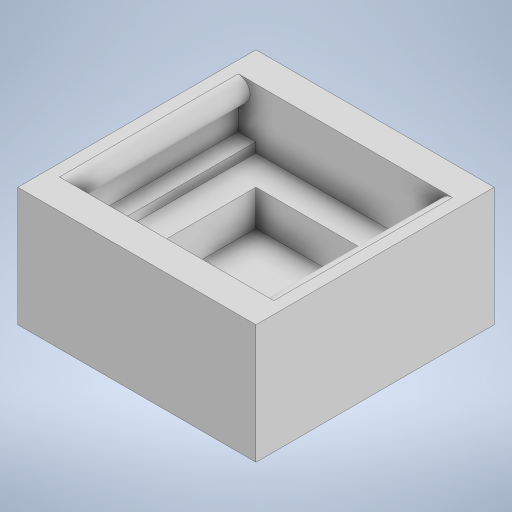
# Autodesk Inventor part: boxtest
Saved by Autodesk Inventor 2023 (Build 270158000, 158)
## iProperties
Created: 2022-12-05
Part Number: boxtest
Material: Generic
Document SubType Name: Modeling
Designer: spfow
Density: 1 g/cm^3
Appearance: Default
Author: spfow
Autodesk Inventor part; units mm, degrees
ref_plane "YZ Plane" through (0, 0, 0) normal (1, 0, 0) x (0, 1, 0)
sketch "Sketch1" plane through (0, 0, 0) normal (0, 1, 0) x (-1, 0, 0)
  line L0 (0, 0) -> (25.4, 0)
  line L1 (25.4, 0) -> (25.4, -25.4)
  line L2 (25.4, -25.4) -> (0, -25.4)
  line L3 (0, -25.4) -> (0, 0)
  dimension "d0" = 25.4
  dimension "d1" = 25.4
  constraints: 8 end point, 2 parallel, 1 horizontal, 1 perpendicular
  measures "d0" distance of L1.end L2.end
  measures "d1" distance of L0.end L1.end
extrude "Extrusion1" add sketch "Sketch1" along normal blind 12.7
shell "Shell1" thickness 6.35 removed faces 1 at (-8.4667, 12.7, -8.4667)
sketch "Sketch2" plane through (0, 12.7, 0) normal (0, 1, 0) x (1, 0, 0)
  line L0 (-22.225, 22.225) -> (-3.175, 22.225)
  line L1 (-3.175, 22.225) -> (-3.175, 3.175)
  line L2 (-3.175, 3.175) -> (-22.225, 3.175)
  line L3 (-22.225, 3.175) -> (-22.225, 22.225)
  line L4 (0, 0) -> (0, 25.4) projected
  line L5 (0, 25.4) -> (-25.4, 25.4) projected
  line L6 (-19.05, 19.05) -> (-6.35, 19.05) projected
  line L7 (-6.35, 19.05) -> (-6.35, 6.35) projected
  line L8 (-19.05, 19.05) -> (-6.35, 19.05)
  line L9 (-6.35, 19.05) -> (-6.35, 6.35)
  line L10 (-6.35, 6.35) -> (-19.05, 6.35)
  line L11 (-19.05, 6.35) -> (-19.05, 19.05)
  dimension "d5" = 19.05
  dimension "d6" = 19.05
  dimension "d7" = 3.175
  dimension "d8" = 3.175
  constraints: 16 end point, 4 parallel, 2 horizontal, 2 perpendicular
  measures "d5" distance of L0.start L0.end
  measures "d6" distance of L0.end L1.end
  measures "d7" distance between parallel lines of L4 L1
  measures "d8" distance between parallel lines of L5 L0
extrude "Extrusion2" cut sketch "Sketch2" against normal blind 10.16 contours L6 L7 L10 L11
extrude "Extrusion3" cut sketch "Sketch2" against normal blind 6.35
ref_plane "Work Plane1" through (-25.4, 0, -12.7) normal (0, 0, 1) x (1, 0, 0)
ref_plane "Work Plane2" through (-12.7, 0, 0) normal (1, 0, 0) x (0, 0, -1)
sketch "Sketch3" plane through (-25.4, 0, -12.7) normal (0, 0, 1) x (1, 0, 0)
  line L0 (25.4, 12.7) -> (0, 12.7) projected
  circle A0 centre (1.27, 11.43) radius 1.27
  line L1 (0, 0) -> (0, 12.7) projected
  circle A1 centre (24.13, 11.43) radius 1.27
  line L2 (25.4, 0) -> (25.4, 12.7) projected
  line L3 (0, 12.7) -> (1.27, 12.7)
  line L4 (1.27, 12.7) -> (1.27, 7.366)
  line L5 (1.27, 7.366) -> (0, 7.366)
  line L6 (0, 7.366) -> (0, 12.7)
  line L7 (0, 12.7) -> (3.81, 12.7)
  line L8 (3.81, 12.7) -> (3.81, 7.366)
  line L9 (3.81, 7.366) -> (0, 7.366)
  line L10 (0, 7.366) -> (0, 12.7)
  line L11 (25.4, 0) -> (25.4, 12.7) projected
  line L12 (25.4, 12.7) -> (24.13, 12.7)
  line L13 (24.13, 12.7) -> (24.13, 7.366)
  line L14 (24.13, 7.366) -> (25.4, 7.366)
  line L15 (25.4, 7.366) -> (25.4, 12.7)
  line L16 (25.4, 12.7) -> (21.59, 12.7)
  line L17 (21.59, 12.7) -> (21.59, 7.366)
  line L18 (21.59, 7.366) -> (25.4, 7.366)
  line L19 (25.4, 7.366) -> (25.4, 12.7)
  point P0 (24.13, 10.16)
  point P1 (24.13, 12.7)
  point P2 (1.27, 7.366)
  point P3 (3.81, 12.7)
  point P4 (1.27, 12.7)
  point P5 (1.27, 10.16)
  dimension "d16" = 2.54
  dimension "d17" = 1.27
  dimension "d18" = 1.27
  dimension "d20" = 2.54
  dimension "d21" = 1.27
  dimension "d22" = 1.27
  dimension "d23" = 1.27
  dimension "d24" = 5.334
  dimension "d25" = 1.27
  dimension "d26" = 5.334
  dimension "d27" = 3.81
  dimension "d28" = 5.334
  dimension "d29" = 5.334
  dimension "d30" = 3.81
  constraints: 32 end point, 8 parallel, 4 horizontal, 4 perpendicular, 2 centre point
  measures "d16" diameter of A0
  measures "d17" distance from line of L0 A0.centre
  measures "d18" distance from line of L1 A0.centre
  measures "d20" diameter of A1
  measures "d21" distance from line of L0 A1.centre
  measures "d22" distance from line of L2 A1.centre
  measures "d23" distance of L4.end L5.end
  measures "d24" distance of L3.end L4.end
  measures "d25" distance of L14.end L13.end
  measures "d26" distance of L12.end L13.end
  measures "d27" distance of L18.end L17.end
  measures "d28" distance of L16.end L17.end
  measures "d29" distance of L7.end L8.end
  measures "d30" distance of L8.end L9.end
extrude "Extrusion4" cut sketch "Sketch3" along normal mid plane 19.05 contours L8 L9 L4 A0 L0 | A1 L13 L18 L17 L0
sketch "Sketch4" plane through (-12.7, 0, 0) normal (1, 0, 0) x (0, 0, -1)
  circle A0 centre (1.27, 11.43) radius 1.27
  circle A1 centre (24.13, 11.43) radius 1.27
  line L0 (0, 12.7) -> (25.4, 12.7) projected
  line L1 (25.4, 0) -> (25.4, 12.7) projected
  line L2 (0, 0) -> (0, 12.7) projected
  line L3 (0, 12.7) -> (1.27, 12.7)
  line L4 (1.27, 12.7) -> (1.27, 8.89)
  line L5 (1.27, 8.89) -> (0, 8.89)
  line L6 (0, 8.89) -> (0, 12.7)
  line L7 (25.4, 12.7) -> (24.13, 12.7)
  line L8 (24.13, 12.7) -> (24.13, 8.89)
  line L9 (24.13, 8.89) -> (25.4, 8.89)
  line L10 (25.4, 8.89) -> (25.4, 12.7)
  line L11 (0, 12.7) -> (3.81, 12.7)
  line L12 (3.81, 12.7) -> (3.81, 8.89)
  line L13 (3.81, 8.89) -> (0, 8.89)
  line L14 (0, 8.89) -> (0, 12.7)
  line L15 (25.4, 12.7) -> (21.59, 12.7)
  line L16 (21.59, 12.7) -> (21.59, 8.89)
  line L17 (21.59, 8.89) -> (25.4, 8.89)
  line L18 (25.4, 8.89) -> (25.4, 12.7)
  dimension "d33" = 2.54
  dimension "d34" = 2.54
  dimension "d35" = 1.27
  dimension "d36" = 1.27
  dimension "d37" = 1.27
  dimension "d38" = 1.27
  dimension "d39" = 1.27
  dimension "d40" = 3.81
  dimension "d41" = 1.27
  dimension "d42" = 3.81
  dimension "d43" = 3.81
  dimension "d44" = 3.81
  dimension "d45" = 3.81
  dimension "d46" = 3.81
  constraints: 32 end point, 8 parallel, 4 horizontal, 4 perpendicular, 2 centre point, 1 point on line
  measures "d33" diameter of A0
  measures "d34" diameter of A1
  measures "d35" distance from line of L0 A1.centre
  measures "d36" distance from line of L1 A1.centre
  measures "d37" distance from line of L0 A0.centre
  measures "d38" distance from line of L2 A0.centre
  measures "d39" distance of L4.end L5.end
  measures "d40" distance of L3.end L4.end
  measures "d41" distance of L9.end L8.end
  measures "d42" distance of L7.end L8.end
  measures "d43" distance of L12.end L13.end
  measures "d44" distance of L17.end L16.end
  measures "d45" distance of L11.end L12.end
  measures "d46" distance of L15.end L16.end
body "Solid1"
